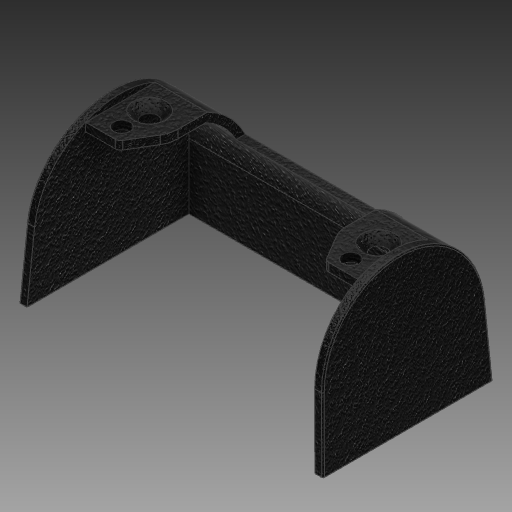
# Autodesk Inventor part: OSŁONA MECHANIZMU PRZECHYLANIA MONITORA
Saved by Autodesk Inventor 2017 SP1 (Build 210196100, 196)
## iProperties
Created: 2021-01-02
Part Number: OSŁONA MECHANIZMU PRZECHYLANIA MONITORA
Material: Tworzywo sztuczne, nieprzezroczyste czarne
Document SubType Name: Modeling
Designer: Napoleon
Density: 0.952 g/cm^3
Appearance: Chropowaty, teksturowany - czarny
Mass: 3.95807 g
Surface Area: 60.1575 cm^2
Volume: 4.15764 cm^3
Author: Napoleon
Autodesk Inventor part; units mm, degrees
ref_plane "YZ Plane" through (0, 0, 0) normal (1, 0, 0) x (0, 1, 0)
ref_plane "XZ Plane" through (0, 0, 0) normal (0, 1, 0) x (-1, 0, 0)
ref_plane "XY Plane" through (0, 0, 0) normal (0, 0, 1) x (1, 0, 0)
sketch "Szkic2" plane through (0, 0, 0) normal (1, 0, 0) x (0, 1, 0)
  line L0 (0, -31.3) -> (0, 0)
  line L1 (0, 0) -> (12.785649, -0.670589)
  line L2 (0, -31.3) -> (12.785649, -30.629411)
  arc A0 (12.785649, -30.629411) -> (12.785649, -0.670589) centre (12, -15.65) ccw
  dimension "d88" = 15
  constraints: 6 end point, 2 point on circle, 1 centre point, 1 tangent
  measures "d88" radius of A0
extrude "Wyciągnięcie proste1" add sketch "Szkic2" along normal blind 56
shell "Skorupa1" thickness 1.5 removed faces 1 at (18.666667, 0, -10.433333)
ref_plane "Płaszczyzna konstrukcyjna3" through (56, 0, 0) normal (0, 0, 1) x (1, 0, 0)
sketch "Szkic5" plane through (56, 0, 0) normal (0, 0, 1) x (1, 0, 0)
  line L0 (-54.5, 27) -> (-54.5, 25.5)
  line L1 (-12.5, 18.5) -> (-43.5, 18.5)
  line L2 (-54.5, 25.5) -> (-43.5, 25.5)
  line L3 (-43.5, 18.5) -> (-43.5, 25.5)
  line L4 (-1.5, 27) -> (-1.5, 25.5)
  line L5 (-1.5, 25.5) -> (-12.5, 25.5)
  line L6 (-12.5, 18.5) -> (-12.5, 25.5)
  line L7 (-54.5, 27) -> (-1.5, 27)
  constraints: 16 end point, 1 horizontal, 1 perpendicular
extrude "Wyciągnięcie proste3" cut sketch "Szkic5" against normal through all
sketch "Szkic6" plane through (1.5, 0, -1.502062) normal (1, 0, 0) x (0, 0, -1)
  arc A0 (7.897938, 23.966098) -> (0.666468, 12.707084) centre (14.147938, 12) ccw
  line L0 (0.666468, 12.707084) -> (0, 0)
  line L1 (7.897938, 25.5) -> (7.60959, 25.5)
  arc A1 (7.60959, 25.5) -> (-0.831473, 12.785649) centre (14.147938, 12) ccw
  line L2 (7.897938, 25.5) -> (7.897938, 23.966098)
  line L3 (-0.831473, 12.785649) -> (-1.502062, 0)
  line L4 (-0.831473, 12.785649) -> (-1.502062, 0)
  line L5 (-1.502062, 0) -> (0, 0)
  line L6 (28.295877, 0) -> (0, 0)
  line L7 (28.295877, 0) -> (27.629408, 12.707084)
  arc A2 (27.629408, 12.707084) -> (14.147938, 25.5) centre (14.147938, 12) ccw
  arc A3 (14.147938, 25.5) -> (0.666468, 12.707084) centre (14.147938, 12) ccw
  line L8 (0.666468, 12.707084) -> (0, 0)
  constraints: 12 end point, 4 point on circle, 2 centre point, 1 collinear, 1 horizontal
extrude "Wyciągnięcie proste4" cut sketch "Szkic6" along normal up to surface (53 mm away) contours A0 L0 L5 L3 A1 L1 L2
sketch "Szkic7" plane through (12.5, 23.966098, -9.4) normal (1, 0, 0) x (0, 0, -1)
  line L0 (0, 0) -> (12.5, 0)
  arc A0 (12.5, 0) -> (6.25, 1.533902) centre (6.25, -11.966098) ccw
  arc A1 (6.25, 1.533902) -> (0, 0) centre (6.25, -11.966098) ccw
  point P0 (-9.4, -23.966098)
  constraints: 4 point on circle, 2 centre point, 2 end point, 1 horizontal
extrude "Wyciągnięcie proste5" add sketch "Szkic7" against normal up to surface (11 mm away)
sketch "Szkic8" plane through (43.5, 23.966098, -9.4) normal (-1, 0, 0) x (0, 0, 1)
  arc A0 (0, 0) -> (-6.25, 1.533902) centre (-6.25, -11.966098) ccw
  arc A1 (-6.25, 1.533902) -> (-12.5, 0) centre (-6.25, -11.966098) ccw
  line L0 (0, 0) -> (-12.5, 0)
  point P0 (9.4, -23.966098)
  constraints: 4 point on circle, 2 centre point, 2 end point
extrude "Wyciągnięcie proste6" add sketch "Szkic8" against normal up to surface (11 mm away)
sketch "Szkic10" plane through (1.5, 25.5, -9.4) normal (0, 0, 1) x (1, 0, 0)
  line L0 (-1.5, -25.5) -> (0, -25.5)
  line L1 (0, 1.5) -> (-1.5, -25.5)
  line L2 (-1.5, -25.5) -> (0, 1.5)
  line L3 (0, 1.5) -> (1.5, 1.5)
  line L4 (1.5, 1.5) -> (0, -25.5)
  line L5 (26.5, -25.5) -> (26.5, 0.111111)
  line L6 (54.5, -25.5) -> (53, -25.5)
  line L7 (53, 1.5) -> (54.5, -25.5)
  line L8 (54.5, -25.5) -> (53, 1.5)
  line L9 (53, 1.5) -> (51.5, 1.5)
  line L10 (51.5, 1.5) -> (53, -25.5)
  dimension "d38" = 1.5
  constraints: 22 end point, 4 symmetric about line, 1 collinear, 1 horizontal, 1 vertical
  measures "d38" distance of L1.start L3.end
extrude "Wyciągnięcie proste8" add sketch "Szkic10" against normal up to surface starts on plane at (0, 12.785649, -0.670589) facing (0, 0.0523766, 0.9986274) surface through (0, 0, -31.3) normal (0, 0.0523766, -0.9986274)
sketch "Szkic11" plane through (12.5, 23.966098, -9.4) normal (0, 0, 1) x (1, 0, 0)
  line L0 (-12.5, -23.966098) -> (-12.5, 3.033902)
  line L1 (-12.5, 3.033902) -> (-11, 3.033902)
  line L2 (-12.5, 3.033902) -> (-11, 3.033902) construction
  line L3 (-11, 3.033902) -> (-12.5, -23.966098)
  line L4 (43.5, -23.966098) -> (43.5, 3.033902)
  line L5 (43.5, 3.033902) -> (42, 3.033902)
  line L6 (43.5, 3.033902) -> (42, 3.033902) construction
  line L7 (42, 3.033902) -> (43.5, -23.966098)
  constraints: 16 end point, 1 collinear, 1 horizontal
extrude "Wyciągnięcie proste9" cut sketch "Szkic11" against normal up to surface starts on plane at (0, 12.785649, -0.670589) facing (0, 0.0523766, 0.9986274) surface through (0, 0, -31.3) normal (0, 0.0523766, -0.9986274)
ref_plane "Płaszczyzna konstrukcyjna5" through (-2.5, 18.5, -27.48216) normal (1, 0, 0) x (0, 0, -1)
sketch "Szkic14" plane through (-2.5, 18.5, -27.48216) normal (1, 0, 0) x (0, 0, -1)
  arc A0 (3.147252, -5.714351) -> (-26.811571, -5.714351) centre (-11.83216, -6.5) ccw
  line L0 (-26.811571, -5.714351) -> (-27.811571, -5.714351)
  line L1 (-27.811571, -5.714351) -> (-27.811571, 9.285649)
  line L2 (3.147252, -5.714351) -> (4.147252, -5.714351)
  line L3 (4.147252, -5.714351) -> (4.147252, 9.285649)
  line L4 (4.147252, 9.285649) -> (-27.811571, 9.285649)
  dimension "d56" = 1
  constraints: 10 end point, 2 horizontal, 2 point on circle, 1 centre point, 1 perpendicular
  measures "d56" distance of L0.start L0.end
extrude "Wyciągnięcie proste11" cut sketch "Szkic14" along normal up to surface surface through (54.5, 27, -9.4) normal (0.9984604, 0.05547, 0)
sketch "Szkic15" plane through (12.5, 25.5, -9.4) normal (0, 1, 0) x (1, 0, 0)
  line L0 (0, 0) -> (0, 6)
  line L1 (0, 6) -> (-3.583333, 0)
  line L2 (-3.583333, 0) -> (0, 0)
  line L3 (31, 0) -> (31, 6)
  line L4 (31, 6) -> (34.583333, 0)
  line L5 (34.583333, 0) -> (31, 0)
  circle A0 centre (-5.583333, 2.625) radius 1.5
  circle A1 centre (36.583333, 2.625) radius 1.5
  line L6 (-9.583333, 12.788348) -> (-9.583333, 0)
  line L7 (-9.583333, 0) -> (0, 0)
  line L8 (31, 0) -> (0, 0)
  line L9 (40.583333, 0) -> (40.583333, 12.788348)
  point P0 (11.083333, 0)
  dimension "d84" = 2.625
  dimension "d85" = 2.625
  dimension "d86" = 4
  dimension "d87" = 4
  constraints: 12 end point, 2 centre point, 1 horizontal
  measures "d84" distance from line of L7 A0.centre
  measures "d85" distance from line of L8 A1.centre
  measures "d86" distance from line of L6 A0.centre
  measures "d87" distance from line of L9 A1.centre
extrude "Wyciągnięcie proste12" cut sketch "Szkic15" against normal through all
sketch "Szkic16" plane through (2.916667, 25.5, -22.188348) normal (0, 1, 0) x (1, 0, 0)
  point P0 (-2.916667, -22.188348)
  point P1 (4, -5.038348)
  point P2 (46.166667, -5.038348)
hole "Otwór1" at (6.916667, 25.5, -17.15) at (49.083333, 25.5, -17.15) direction (0, -1, 0) diameter 3 end through all countersink diameter 6 countersink angle 90
fillet "Zaokrąglenie1" radius 0.25 8 edges at (54.7288, 22.8808, -25.9751) (54.7288, 22.8808, -5.3249) (55.6448, 6.3928, -30.9647) (55.6448, 6.3928, -0.3353) (1.2712, 22.8808, -5.3249) (1.2712, 22.8808, -25.9751) (0.3552, 6.3928, -30.9647) (0.3552, 6.3928, -0.3353)
fillet "Zaokrąglenie2" radius 5 2 edges at (12.5, 24.733, -15.4) (43.5, 24.733, -15.4)
fillet "Zaokrąglenie3" radius 1 2 edges at (8.9167, 24.733, -9.4) (47.0833, 24.733, -9.4)
